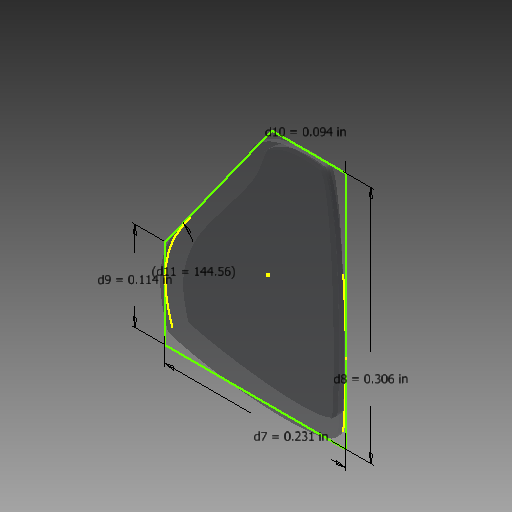
# Autodesk Inventor part: MBS D WINDOW OUTLINE
Saved by Autodesk Inventor 2018.3 (Build 223284000, 284)
## iProperties
Created: 2015-09-03
Material: GLASS, BOROSILICATE
Vendor: HHMI: JRC - ID&F
Document SubType Name: Modeling
Designer: ARNOLDJ
Density: 2.23 g/cm^3
Appearance: Glass
RuleStatus: InUse
AfterDocSave0: file://Part Number Cleaner
DESIGN DEPARTMENT: HHMI: JRC - ID&F
ALTERED ITEM PART NUMBER: N/A
ALTERED ITEM VENDOR: N/A
ALTERED ITEM DESCRIPTION: N/A
Revision Number: 0
Autodesk Inventor part; units mm, degrees
ref_plane "YZ Plane" through (0, 0, 0) normal (1, 0, 0) x (0, 1, 0)
ref_plane "XZ Plane" through (0, 0, 0) normal (0, 1, 0) x (-1, 0, 0)
sketch "Sketch1-Imported DXF File" plane through (0, 0, 0) normal (0, 0, 1) x (1, 0, 0)
  spline S0 degree 3 poles (-0.1804, 3.3652) (0.3809, 3.8577) (0.9425, 3.8911) (1.6669, 3.8045) knots 0 0 0 0 1 1 1 1
  line L0 (-0.1804, 3.3652) -> (0.3809, 3.8577) construction
  line L1 (0.3809, 3.8577) -> (0.9425, 3.8911) construction
  line L2 (0.9425, 3.8911) -> (1.6669, 3.8045) construction
  spline S1 degree 3 poles (1.6669, 3.8045) (2.052, 3.7584) (2.2228, -0.9315) (2.0861, -2.907) knots 1 1 1 1 2 2 2 2
  line L3 (1.6669, 3.8045) -> (2.052, 3.7584) construction
  line L4 (2.052, 3.7584) -> (2.2228, -0.9315) construction
  line L5 (2.2228, -0.9315) -> (2.0861, -2.907) construction
  spline S2 degree 3 poles (2.0861, -2.907) (2.0239, -3.807) (-2.7213, -2.918) (-2.7718, -2.7684) knots 2 2 2 2 3 3 3 3
  line L6 (2.0861, -2.907) -> (2.0239, -3.807) construction
  line L7 (2.0239, -3.807) -> (-2.7213, -2.918) construction
  line L8 (-2.7213, -2.918) -> (-2.7718, -2.7684) construction
  spline S3 degree 3 poles (-2.7718, -2.7684) (-3.6279, -0.2341) (-0.832, 1.069) (-0.1804, 3.3652) knots 3 3 3 3 4 4 4 4
  line L9 (-2.7718, -2.7684) -> (-3.6279, -0.2341) construction
  line L10 (-3.6279, -0.2341) -> (-0.832, 1.069) construction
  line L11 (-0.832, 1.069) -> (-0.1804, 3.3652) construction
  spline S4 degree 3 poles (-0.2918, 3.6041) (0.022, 3.8725) (0.2642, 4.0092) (0.6288, 4.0765) knots 0 0 0 0 1 1 1 1
  line L12 (-0.2918, 3.6041) -> (0.022, 3.8725) construction
  line L13 (0.022, 3.8725) -> (0.2642, 4.0092) construction
  line L14 (0.2642, 4.0092) -> (0.6288, 4.0765) construction
  spline S5 degree 3 poles (0.6288, 4.0765) (0.9935, 4.1434) (1.4802, 4.1406) (1.8853, 4.0933) knots 1 1 1 1 2 2 2 2
  line L15 (0.6288, 4.0765) -> (0.9935, 4.1434) construction
  line L16 (0.9935, 4.1434) -> (1.4802, 4.1406) construction
  line L17 (1.4802, 4.1406) -> (1.8853, 4.0933) construction
  spline S6 degree 3 poles (1.8853, 4.0933) (2.1007, 4.068) (2.348, 2.7989) (2.4228, 1.2572) knots 2 2 2 2 3 3 3 3
  line L18 (1.8853, 4.0933) -> (2.1007, 4.068) construction
  line L19 (2.1007, 4.068) -> (2.348, 2.7989) construction
  line L20 (2.348, 2.7989) -> (2.4228, 1.2572) construction
  spline S7 degree 3 poles (2.4228, 1.2572) (2.5251, -0.8485) (2.5466, -1.4274) (2.4229, -3.1671) knots 3 3 3 3 4 4 4 4
  line L21 (2.4228, 1.2572) -> (2.5251, -0.8485) construction
  line L22 (2.5251, -0.8485) -> (2.5466, -1.4274) construction
  line L23 (2.5466, -1.4274) -> (2.4229, -3.1671) construction
  spline S8 degree 3 poles (2.4229, -3.1671) (2.3865, -3.6579) (0.7942, -3.6867) (-0.6024, -3.5533) knots 4 4 4 4 5 5 5 5
  line L24 (2.4229, -3.1671) -> (2.3865, -3.6579) construction
  line L25 (2.3865, -3.6579) -> (0.7942, -3.6867) construction
  line L26 (0.7942, -3.6867) -> (-0.6024, -3.5533) construction
  spline S9 degree 3 poles (-0.6024, -3.5533) (-1.9971, -3.4205) (-3.0918, -3.117) (-3.1201, -3.0352) knots 5 5 5 5 6 6 6 6
  line L27 (-0.6024, -3.5533) -> (-1.9971, -3.4205) construction
  line L28 (-1.9971, -3.4205) -> (-3.0918, -3.117) construction
  line L29 (-3.0918, -3.117) -> (-3.1201, -3.0352) construction
  spline S10 degree 3 poles (-3.1201, -3.0352) (-3.5986, -1.6526) (-3.3227, -0.6417) (-2.5373, 0.3639) knots 6 6 6 6 7 7 7 7
  line L30 (-3.1201, -3.0352) -> (-3.5986, -1.6526) construction
  line L31 (-3.5986, -1.6526) -> (-3.3227, -0.6417) construction
  line L32 (-3.3227, -0.6417) -> (-2.5373, 0.3639) construction
  spline S11 degree 3 poles (-2.5373, 0.3639) (-2.5757, 0.3147) (-0.3637, 3.3574) (-0.2918, 3.6041) knots 7 7 7 7 8 8 8 8
  line L33 (-2.5373, 0.3639) -> (-2.5757, 0.3147) construction
  line L34 (-2.5757, 0.3147) -> (-0.3637, 3.3574) construction
  line L35 (-0.3637, 3.3574) -> (-0.2918, 3.6041) construction
  point P0 (0, 0)
  constraints: 36 other
sketch "Sketch2" plane through (0, 0, 0) normal (0, 0, 1) x (1, 0, 0)
  spline S0 degree 3 poles (-2.5373, 0.3639) (-1.6488, 1.609) (-0.4725, 3.2194) (-0.2918, 3.6041) knots 0 0 0 0 1 1 1 1
  spline S1 degree 4 poles (-0.2918, 3.6041) (-0.1205, 3.7459) (-0.0329, 3.81) (0.1033, 3.8971) (0.3083, 3.9925) (0.4387, 4.0359) (0.5464, 4.0612) (0.6288, 4.0765) knots 0 0 0 0 0 0.40557 0.536324 0.666446 1 1 1 1 1
  spline S2 degree 4 poles (0.6288, 4.0765) (0.9071, 4.1274) (1.236, 4.141) (1.575, 4.1295) (1.8853, 4.0933) knots 0 0 0 0 0 1 1 1 1 1
  spline S3 degree 4 poles (1.8853, 4.0933) (1.9276, 4.0877) (1.9882, 4.0171) (2.0671, 3.8369) (2.1609, 3.4899) (2.2808, 2.8848) (2.3582, 2.2428) (2.4023, 1.6844) (2.4228, 1.2572) knots 0 0 0 0 0 0.177655 0.283389 0.412601 0.562831 1 1 1 1 1
  spline S4 degree 2 poles (2.4228, 1.2572) (2.593, -1.164) (2.4229, -3.1671) knots 0 0 0 1 1 1
  spline S5 degree 4 poles (2.4229, -3.1671) (2.4172, -3.2595) (2.3276, -3.3767) (2.0958, -3.4872) (1.6709, -3.5741) (1.0134, -3.6358) (0.3511, -3.6264) (-0.2019, -3.5916) (-0.6024, -3.5533) knots 0 0 0 0 0 0.212151 0.321828 0.449986 0.594733 1 1 1 1 1
  spline S6 degree 4 poles (-0.6024, -3.5533) (-0.978, -3.5176) (-1.4691, -3.4535) (-2.0388, -3.3544) (-2.5835, -3.2276) (-2.8889, -3.1434) (-3.048, -3.0858) (-3.1131, -3.0522) (-3.1201, -3.0352) knots 0 0 0 0 0 0.445751 0.600467 0.733494 0.840359 1 1 1 1 1
  spline S7 degree 4 poles (-3.1201, -3.0352) (-3.2285, -2.7218) (-3.3346, -2.3022) (-3.3861, -1.7902) (-3.3167, -1.2009) (-3.1666, -0.6409) (-2.9464, -0.2048) (-2.7224, 0.1268) (-2.5373, 0.3639) knots 0 0 0 0 0 0.32417 0.44647 0.56674 0.687368 1 1 1 1 1
  point P0 (0, 0)
  point P1 (-1.292, 2.1047)
  point P2 (-0.5022, 3.2501)
  point P3 (-0.0522, 3.7921)
  point P4 (0.0556, 3.8626)
  point P5 (0.161, 3.9217)
  point P6 (0.2674, 3.9714)
  point P7 (0.3783, 4.0131)
  point P8 (0.4974, 4.0479)
  point P9 (0.9057, 4.1126)
  point P10 (1.2248, 4.1276)
  point P11 (1.5614, 4.1204)
  point P12 (1.9311, 4.07)
  point P13 (1.9884, 3.9938)
  point P14 (2.0595, 3.8309)
  point P15 (2.1406, 3.5531)
  point P16 (2.2254, 3.1463)
  point P17 (2.3061, 2.6141)
  point P18 (2.3745, 1.9749)
  point P19 (2.5077, -1.1636)
  point P20 (2.3812, -3.282)
  point P21 (2.2671, -3.3858)
  point P22 (2.057, -3.4798)
  point P23 (1.7287, -3.556)
  point P24 (1.2755, -3.6054)
  point P25 (0.7111, -3.6217)
  point P26 (0.0687, -3.6033)
  point P27 (-1.2291, -3.4803)
  point P28 (-1.7932, -3.3917)
  point P29 (-2.2714, -3.2978)
  point P30 (-2.6442, -3.2091)
  point P31 (-2.9004, -3.1353)
  point P32 (-3.0452, -3.0825)
  point P33 (-3.1053, -3.051)
  point P34 (-3.2685, -2.516)
  point P35 (-3.343, -2.0448)
  point P36 (-3.3527, -1.6099)
  point P37 (-3.3039, -1.2004)
  point P38 (-3.1992, -0.8068)
  point P39 (-3.0385, -0.4203)
  point P40 (-2.8193, -0.0327)
  constraints: 56 other
extrude "Extrusion1-Larger Window" add sketch "Sketch2" along normal blind 0.15
sketch "Sketch3" plane through (0, 0, 0) normal (0, 0, 1) x (1, 0, 0)
  spline S0 degree 4 poles (-2.7718, -2.7684) (-2.9175, -2.2324) (-3.0654, -1.6105) (-2.6833, -0.5765) (-2.0778, 0.4174) (-0.2063, 2.7122) (-0.5864, 2.4953) (-0.1804, 3.3652) knots 0 0 0 0 0 0.323574 0.472009 0.62378 1 1 1 1 1
  spline S1 degree 4 poles (-0.1804, 3.3652) (-0.0582, 3.4724) (0.1156, 3.598) (0.3471, 3.7164) (0.6472, 3.8004) (0.9667, 3.849) (1.2484, 3.8466) (1.4846, 3.8262) (1.6669, 3.8045) knots 0 0 0 0 0 0.310542 0.430474 0.550556 0.673226 1 1 1 1 1
  spline S2 degree 4 poles (1.6669, 3.8045) (1.753, 3.7839) (1.8418, 3.5031) (1.9497, 2.8772) (2.0432, 1.772) (2.1286, 0.1628) (2.1456, -1.2825) (2.1266, -2.3145) (2.0861, -2.907) knots 0 0 0 0 0 0.191178 0.313183 0.458164 0.615426 1 1 1 1 1
  spline S3 degree 4 poles (2.0861, -2.907) (2.0814, -2.9893) (2.0169, -3.0937) (1.8459, -3.1913) (1.5284, -3.2661) (1.1923, -3.3011) (0.7723, -3.3097) (0.275, -3.2892) (-0.2688, -3.2444) (-0.8928, -3.1666) (-1.4631, -3.0854) (-2.4303, -2.9022) (-2.7344, -2.812) (-2.7718, -2.7684) knots 0 0 0 0 0 0.121837 0.181897 0.251545 0.330741 0.418194 0.511774 0.608711 0.713595 0.815227 1 1 1 1 1
  point P0 (0, 0)
  point P1 (0.0266, 3.5263)
  point P2 (0.2302, 3.6471)
  point P3 (0.435, 3.7348)
  point P4 (0.6457, 3.7943)
  point P5 (0.8675, 3.8291)
  point P6 (1.1063, 3.8415)
  point P7 (1.3693, 3.8329)
  point P8 (1.737, 3.7424)
  point P9 (1.8285, 3.4825)
  point P10 (1.9312, 2.8876)
  point P11 (2.0254, 1.9214)
  point P12 (2.0951, 0.6699)
  point P13 (2.1298, -0.6901)
  point P14 (2.1256, -1.9444)
  point P15 (2.0516, -3.0154)
  point P16 (1.9634, -3.1075)
  point P17 (1.8086, -3.1872)
  point P18 (1.5702, -3.2508)
  point P19 (1.2383, -3.2915)
  point P20 (0.813, -3.3041)
  point P21 (0.3073, -3.2867)
  point P22 (-0.2547, -3.2408)
  point P23 (-0.8389, -3.1716)
  point P24 (-1.4037, -3.0874)
  point P25 (-2.3015, -2.9158)
  point P26 (-2.71, -2.8043)
  point P27 (-2.9305, -1.9534)
  point P28 (-2.8622, -1.2244)
  point P29 (-2.6092, -0.5289)
  point P30 (-2.1892, 0.1783)
  point P31 (-0.9618, 1.8213)
  point P32 (-0.4934, 2.5857)
  constraints: 40 other
extrude "Extrusion2" add sketch "Sketch3" against normal blind 0.17
ref_plane "Work Plane1" through (0, 0, -0.175) normal (0, 0, -1) x (-1, 0, 0)
sketch "Sketch4" plane through (0, 0, -0.175) normal (0, 0, -1) x (-1, 0, 0)
  spline S0 degree 4 poles (2.7718, -2.7684) (2.9175, -2.2324) (3.0654, -1.6105) (2.6833, -0.5765) (2.0778, 0.4174) (0.2063, 2.7122) (0.5864, 2.4953) (0.1804, 3.3652) knots 0 0 0 0 0 0.323574 0.472009 0.62378 1 1 1 1 1 projected
  spline S1 degree 4 poles (0.1804, 3.3652) (0.0582, 3.4724) (-0.1156, 3.598) (-0.3471, 3.7164) (-0.6472, 3.8004) (-0.9667, 3.849) (-1.2484, 3.8466) (-1.4846, 3.8262) (-1.6669, 3.8045) knots 0 0 0 0 0 0.310542 0.430474 0.550556 0.673226 1 1 1 1 1 projected
  spline S2 degree 4 poles (-1.6669, 3.8045) (-1.753, 3.7839) (-1.8418, 3.5031) (-1.9497, 2.8772) (-2.0432, 1.772) (-2.1286, 0.1628) (-2.1456, -1.2825) (-2.1266, -2.3145) (-2.0861, -2.907) knots 0 0 0 0 0 0.191178 0.313183 0.458164 0.615426 1 1 1 1 1 projected
  spline S3 degree 4 poles (-2.0861, -2.907) (-2.0814, -2.9893) (-2.0169, -3.0937) (-1.8459, -3.1913) (-1.5284, -3.2661) (-1.1923, -3.3011) (-0.7723, -3.3097) (-0.275, -3.2892) (0.2688, -3.2444) (0.8928, -3.1666) (1.4631, -3.0854) (2.4303, -2.9022) (2.7344, -2.812) (2.7718, -2.7684) knots 0 0 0 0 0 0.121837 0.181897 0.251545 0.330741 0.418194 0.511774 0.608711 0.713595 0.815227 1 1 1 1 1 projected
  point P0 (0, 0)
  constraints: 4 other
extrude "Extrusion3" add sketch "Sketch4" along normal blind 0.17
sketch "Sketch5" plane through (0, 0, 0) normal (0, 0, 1) x (1, 0, 0)
  line L0 (-3.3583, -0.7328) -> (-3.3583, -3.6344)
  line L1 (2.5057, -3.6344) -> (2.5057, 4.1337)
  line L2 (0.1055, 4.1337) -> (2.5057, 4.1337)
  line L3 (-3.3583, -3.6344) -> (2.5057, -3.6344)
  line L4 (-3.3583, -0.7328) -> (0.1055, 4.1337)
  point P0 (0, 0)
  dimension "d7" = 5.864
  dimension "d8" = 7.7681
  dimension "d9" = 2.9016
  dimension "d10" = 2.4002
  dimension "d11" = 144.558
  constraints: 10 end point, 2 horizontal, 2 vertical, 2 other
  measures "d7" distance between parallel lines of L1 L0
  measures "d8" distance between parallel lines of L3 L2
  measures "d9" distance of L0.start L0.end
  measures "d10" distance of L2.start L1.end
  measures "d11" angle of L0 L4
body "Solid1"
